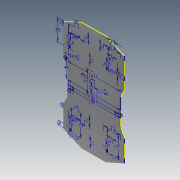
# Autodesk Inventor part: podvozek_+_prametry
Saved by Autodesk Inventor 2013 (Build 170138000, 138)
## iProperties
Created: 2012-08-22
Part Number: podvozek_+_prametry
Material: Generic
Document SubType Name: Modeling
Designer: idle-rug
Density: 1 g/cm^3
Author: idle-rug
Autodesk Inventor part; units mm, degrees
ref_plane "YZ Plane" through (0, 0, 0) normal (1, 0, 0) x (0, 1, 0)
ref_plane "XZ Plane" through (0, 0, 0) normal (0, 1, 0) x (-1, 0, 0)
ref_plane "XY Plane" through (0, 0, 0) normal (0, 0, 1) x (1, 0, 0)
sketch "Sketch1" plane through (0, 0, 0) normal (0, 1, 0) x (-1, 0, 0)
  line L0 (-75.5, -115.65) -> (-75.5, -62.65)
  line L1 (-65.5, -42.65) -> (-75.5, -62.65)
  line L2 (75.5, -115.65) -> (75.5, -62.65)
  line L3 (65.5, -42.65) -> (75.5, -62.65)
  line L4 (-75.5, 115.65) -> (-75.5, 42.15)
  line L5 (-65.5, 22.15) -> (-75.5, 42.15)
  line L6 (75.5, 115.65) -> (75.5, 42.15)
  line L7 (65.5, 22.15) -> (75.5, 42.15)
  line L8 (30.5, 135.65) -> (75.5, 115.65)
  line L9 (-30.5, 135.65) -> (-75.5, 115.65)
  line L10 (30.5, -135.65) -> (75.5, -115.65)
  line L11 (-30.5, -135.65) -> (-75.5, -115.65)
  line L12 (65.5, 22.15) -> (65.5, -42.65)
  line L13 (-65.5, -42.65) -> (-65.5, 22.15)
  line L14 (30.5, -135.65) -> (-30.5, -135.65)
  line L15 (30.5, 135.65) -> (-30.5, 135.65)
  constraints: 32 end point, 2 parallel, 1 perpendicular, 1 point on line
extrude "Extrusion1" add sketch "Sketch1" along normal blind 2
sketch "Sketch2" plane through (0, 2, 0) normal (0, 1, 0) x (1, 0, 0)
  line L0 (75.5, 62.65) -> (75.5, 115.65) projected
  line L1 (75.5, 115.65) -> (30.5, 135.65) projected
  line L2 (30.5, 135.65) -> (-30.5, 135.65) projected
  line L3 (-30.5, 135.65) -> (-75.5, 115.65) projected
  line L4 (-75.5, 115.65) -> (-75.5, 62.65) projected
  line L5 (-75.5, 62.65) -> (-65.5, 42.65) projected
  line L6 (-65.5, 42.65) -> (-65.5, -22.15) projected
  line L7 (-65.5, -22.15) -> (-75.5, -42.15) projected
  line L8 (-75.5, -115.65) -> (-30.5, -135.65) projected
  line L9 (-30.5, -135.65) -> (30.5, -135.65) projected
  line L10 (30.5, -135.65) -> (75.5, -115.65) projected
  line L11 (75.5, -115.65) -> (75.5, -42.15) projected
  line L12 (75.5, -42.15) -> (65.5, -22.15) projected
  line L13 (65.5, -22.15) -> (65.5, 42.65) projected
  line L14 (65.5, 42.65) -> (75.5, 62.65) projected
  line L15 (-75.5, -115.65) -> (75.5, -115.65)
  line L16 (-75.5, -42.15) -> (75.5, -42.15)
  line L17 (-75.5, 62.65) -> (75.5, 62.65)
  line L18 (-75.5, 115.65) -> (75.5, 115.65)
  line L19 (-75.5, 115.65) -> (-75.5, 105.65)
  line L20 (-75.5, 105.65) -> (75.5, 105.65)
  line L21 (75.5, 115.65) -> (75.5, 105.65)
  line L22 (-75.5, 62.65) -> (-75.5, 72.65)
  line L23 (-75.5, 72.65) -> (75.5, 72.65)
  line L24 (75.5, 62.65) -> (75.5, 72.65)
  line L25 (-75.5, -115.65) -> (-75.5, -105.65)
  line L26 (-75.5, -105.65) -> (75.5, -105.65)
  line L27 (75.5, -105.65) -> (75.5, -115.65)
  line L28 (-75.5, -62.65) -> (75.5, -62.65)
  line L29 (-65.5, 42.65) -> (-65.5, 120.0944)
  line L30 (65.5, 42.65) -> (65.5, 120.0944)
  line L31 (-65.5, -22.15) -> (-65.5, -120.0944)
  line L32 (65.5, -22.15) -> (65.5, -120.0944)
  line L33 (75.5, -62.65) -> (75.5, -72.65)
  line L34 (75.5, -72.65) -> (-75.5, -72.65)
  line L35 (-75.5, -62.65) -> (-75.5, -72.65)
  line L36 (-75.5, -42.15) -> (-75.5, -115.65)
  line L37 (65.5, -62.65) -> (40.6, -62.65)
  line L38 (40.6, -62.65) -> (40.6, -115.65)
  line L39 (40.6, -115.65) -> (50.6, -115.65)
  line L40 (50.6, -115.65) -> (50.6, -62.65)
  line L41 (50.6, -62.65) -> (40.6, -62.65)
  line L42 (-65.5, -62.65) -> (-40.6, -62.65)
  line L43 (-40.6, -62.65) -> (-40.6, -115.65)
  line L44 (-40.6, -115.65) -> (-50.6, -115.65)
  line L45 (-50.6, -115.65) -> (-50.6, -62.65)
  line L46 (-50.6, -62.65) -> (-40.6, -62.65)
  line L47 (-65.5, 115.65) -> (-40.6, 115.65)
  line L48 (-40.6, 115.65) -> (-40.6, 62.65)
  line L49 (-40.6, 62.65) -> (-50.6, 62.65)
  line L50 (-50.6, 62.65) -> (-50.6, 115.65)
  line L51 (-50.6, 115.65) -> (-40.6, 115.65)
  line L52 (65.5, 115.65) -> (40.6, 115.65)
  line L53 (40.6, 115.65) -> (40.6, 62.65)
  line L54 (40.6, 62.65) -> (50.6, 62.65)
  line L55 (50.6, 62.65) -> (50.6, 115.65)
  line L56 (50.6, 115.65) -> (40.6, 115.65)
  line L57 (-65.5, 12.65) -> (65.5, 12.65)
  line L58 (65.5, 12.65) -> (65.5, 22.65)
  line L59 (65.5, 22.65) -> (-65.5, 22.65)
  line L60 (-65.5, 22.65) -> (-65.5, 12.65)
  line L61 (0, 12.65) -> (0, -42.15)
  line L62 (-65.5, -42.15) -> (-65.5, 5.85)
  line L63 (-65.5, 5.85) -> (65.5, 5.85)
  line L64 (65.5, 5.85) -> (65.5, -42.15)
  line L65 (-65.5, -42.15) -> (-65.5, -40.15)
  line L66 (-65.5, -40.15) -> (65.5, -40.15)
  line L67 (65.5, -40.15) -> (65.5, -42.15)
  circle A0 centre (-70.5, 110.65) radius 1.2
  circle A1 centre (-70.5, 67.65) radius 1.2
  circle A2 centre (70.5, 110.65) radius 1.2
  circle A3 centre (70.5, 67.65) radius 1.2
  line L68 (-65.5, 115.65) -> (-24.1, 115.65)
  line L69 (65.5, 115.65) -> (24.1, 115.65)
  line L70 (-65.5, 72.65) -> (0, 72.65)
  line L71 (0, 22.65) -> (0, 17.65)
  circle A4 centre (0, 17.65) radius 1.2
  line L72 (-65.5, 22.65) -> (-60.5, 22.65)
  line L73 (-60.5, 22.65) -> (-60.5, 17.65)
  circle A5 centre (-60.5, 17.65) radius 1.2
  line L74 (65.5, 22.65) -> (60.5, 22.65)
  line L75 (60.5, 22.65) -> (60.5, 17.65)
  circle A6 centre (60.5, 17.65) radius 1.2
  line L76 (0, 5.85) -> (0, -17.15)
  line L77 (0, -17.15) -> (-32.15, -17.15)
  line L78 (0, -17.15) -> (32.15, -17.15)
  circle A7 centre (-32.15, -17.15) radius 1.2
  circle A8 centre (32.15, -17.15) radius 1.2
  line L79 (75.5, -42.15) -> (70.5, -42.15)
  circle A9 centre (70.5, -42.15) radius 1.2
  circle A10 centre (70.5, -67.65) radius 1.2
  circle A11 centre (70.5, -110.65) radius 1.2
  circle A12 centre (-70.5, -67.65) radius 1.2
  circle A13 centre (-70.5, -110.65) radius 1.2
  line L80 (-75.5, -42.15) -> (-70.5, -42.15)
  circle A14 centre (-70.5, -42.15) radius 1.2
  line L81 (0, -62.65) -> (0, -67.65)
  circle A15 centre (0, -67.65) radius 1.2
  line L82 (0, 115.65) -> (0, 110.65)
  circle A16 centre (0, 110.65) radius 1.2
  line L83 (-65.5, 72.65) -> (-24.1, 72.65)
  line L84 (-24.1, 72.65) -> (-24.1, 67.65)
  line L85 (65.5, 72.65) -> (24.1, 72.65)
  line L86 (24.1, 72.65) -> (24.1, 67.65)
  circle A17 centre (-24.1, 67.65) radius 1.2
  circle A18 centre (24.1, 67.65) radius 1.2
  line L87 (-65.5, -105.65) -> (-24.1, -105.65)
  line L88 (-24.1, -105.65) -> (-24.1, -110.65)
  line L89 (65.5, -105.65) -> (24.1, -105.65)
  line L90 (24.1, -105.65) -> (24.1, -110.65)
  circle A19 centre (-24.1, -110.65) radius 1.2
  circle A20 centre (24.1, -110.65) radius 1.2
  line L91 (-50.6, -62.65) -> (-50.6, -89.15)
  line L92 (-50.6, -89.15) -> (-45.6, -89.15)
  line L93 (40.6, -62.65) -> (40.6, -89.15)
  line L94 (40.6, -89.15) -> (45.6, -89.15)
  line L95 (40.6, 115.65) -> (40.6, 89.15)
  line L96 (40.6, 89.15) -> (45.6, 89.15)
  line L97 (-50.6, 115.65) -> (-50.6, 89.15)
  line L98 (-50.6, 89.15) -> (-45.6, 89.15)
  circle A21 centre (-45.6, 89.15) radius 1.2
  circle A22 centre (45.6, 89.15) radius 1.2
  circle A23 centre (45.6, -89.15) radius 1.2
  circle A24 centre (-45.6, -89.15) radius 1.2
  point P0 (0, 0)
  dimension "d26" = 10
  dimension "d27" = 10
  dimension "d28" = 10
  dimension "d29" = 53
  dimension "d30" = 10
  dimension "d31" = 24.9
  dimension "d32" = 53
  dimension "d33" = 10
  dimension "d35" = 24.9
  dimension "d36" = 10
  dimension "d37" = 53
  dimension "d38" = 24.9
  dimension "d39" = 53
  dimension "d40" = 10
  dimension "d41" = 53
  dimension "d42" = 24.9
  dimension "d43" = 53
  dimension "d44" = 10
  dimension "d45" = 53
  dimension "d47" = 131
  dimension "d48" = 10
  dimension "d49" = 131
  dimension "d50" = 54.8
  dimension "d51" = 48
  dimension "d52" = 131
  dimension "d53" = 2
  dimension "d54" = 131
  dimension "d68" = 5
  dimension "d70" = 5
  dimension "d71" = 5
  dimension "d73" = 5
  dimension "d74" = 5
  dimension "d76" = 23
  dimension "d77" = 32.15
  dimension "d78" = 32.15
  dimension "d86" = 5
  dimension "d88" = 5
  dimension "d90" = 5
  dimension "d92" = 41.4
  dimension "d93" = 5
  dimension "d94" = 41.4
  dimension "d98" = 41.4
  dimension "d99" = 5
  dimension "d100" = 41.4
  dimension "d101" = 5
  dimension "d104" = 26.5
  dimension "d105" = 5
  dimension "d106" = 26.5
  dimension "d107" = 5
  dimension "d108" = 26.5
  dimension "d109" = 5
  dimension "d110" = 26.5
  dimension "d111" = 5
  constraints: 166 end point, 60 point on line, 25 centre point, 23 perpendicular, 17 coincident, 10 midpoint, 9 collinear, 4 parallel, 1 horizontal, 10 other
  measures "d26" distance of L3.end L19.end
  measures "d27" distance of L4.end L22.end
  measures "d28" distance of L8.start L25.end
  measures "d29" distance of L8.start L28.start
  measures "d30" distance of L28.end L33.end
  measures "d31" distance of L37.start L37.end
  measures "d32" distance of L37.end L38.end
  measures "d33" distance of L38.end L39.end
  measures "d35" distance of L42.start L42.end
  measures "d36" distance of L43.end L44.end
  measures "d37" distance of L44.end L45.end
  measures "d38" distance of L47.start L47.end
  measures "d39" distance of L47.end L48.end
  measures "d40" distance of L48.end L49.end
  measures "d41" distance of L49.end L50.end
  measures "d42" distance of L52.start L52.end
  measures "d43" distance of L52.end L53.end
  measures "d44" distance of L53.end L54.end
  measures "d45" distance of L54.end L55.end
  measures "d47" distance of L57.start L57.end
  measures "d48" distance of L57.end L58.end
  measures "d49" distance of L58.end L59.end
  measures "d50" distance of L61.start L61.end
  measures "d51" distance of L62.start L62.end
  measures "d52" distance of L62.end L63.end
  measures "d53" distance of L62.start L65.end
  measures "d54" distance of L65.end L66.end
  measures "d68" distance of L71.start L71.end
  measures "d70" distance of L59.end L72.end
  measures "d71" distance of L72.end L73.end
  measures "d73" distance of L58.end L74.end
  measures "d74" distance of L74.end L75.end
  measures "d76" distance of L76.start L76.end
  measures "d77" distance of L76.end L77.end
  measures "d78" distance of L76.end L78.end
  measures "d86" distance of L7.end L80.end
  measures "d88" distance of L81.start L81.end
  measures "d90" distance of L82.start L82.end
  measures "d92" distance of L70.start L83.end
  measures "d93" distance of L83.end L84.end
  measures "d94" distance of L85.start L85.end
  measures "d98" distance of L87.start L87.end
  measures "d99" distance of L87.end L88.end
  measures "d100" distance of L89.start L89.end
  measures "d101" distance of L89.end L90.end
  measures "d104" distance of L45.end L91.end
  measures "d105" distance of L91.end L92.end
  measures "d106" distance of L37.end L93.end
  measures "d107" distance of L93.end L94.end
  measures "d108" distance of L52.end L95.end
  measures "d109" distance of L95.end L96.end
  measures "d110" distance of L50.end L97.end
  measures "d111" distance of L97.end L98.end
body "Solid1"
